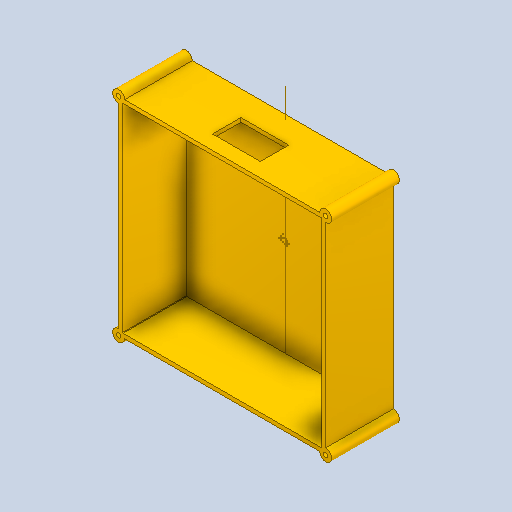
# Autodesk Inventor part: PS-01
Saved by Autodesk Inventor 2022 (Build 260153000, 153)
## iProperties
Company: El Camino College
Created: 2023-06-09
Part Number: PS-01
Material: Aluminum 6061(1)
Document SubType Name: Modeling
Designer: Edgar Tejada
Density: 2.7 g/cm^3
Appearance: Aluminum - Flat(1)
Mass: 533.78 g
Surface Area: 1266.21 cm^2
Volume: 197.696 cm^3
Author: Edgar Tejada
Title: Panel Shell
Autodesk Inventor part; units mm, degrees
ref_plane "YZ Plane" through (0, 0, 0) normal (1, 0, 0) x (0, 1, 0)
ref_plane "XZ Plane" through (0, 0, 0) normal (0, 1, 0) x (-1, 0, 0)
ref_plane "XY Plane" through (0, 0, 0) normal (0, 0, 1) x (1, 0, 0)
sketch "Sketch1" plane through (0, 0, 0) normal (0, 0, 1) x (1, 0, 0)
  line L0 (-79.375, 79.375) -> (79.375, 79.375)
  line L1 (79.375, 79.375) -> (79.375, -79.375)
  line L2 (79.375, -79.375) -> (-79.375, -79.375)
  line L3 (-79.375, -79.375) -> (-79.375, 79.375)
  line L4 (-79.375, 79.375) -> (79.375, -79.375) construction
  line L5 (79.375, 79.375) -> (-79.375, -79.375) construction
  point P0 (0, 0)
  dimension "d0" = 158.75
  constraints: 12 end point, 2 midpoint, 2 parallel, 2 perpendicular, 1 horizontal
  measures "d0" distance of L2.end L0.start
extrude "Extrusion1" add sketch "Sketch1" along normal blind 50.8
shell "Shell1" thickness 3.175 outward yes removed faces 1 at (-26.4583, 26.4583, 50.8)
sketch "Sketch2" plane through (0, 0, 0) normal (0, 0, 1) x (1, 0, 0)
  line L0 (-82.55, 82.55) -> (-82.55, -82.55) projected
  circle A0 centre (-82.55, 82.55) radius 4.7752
  line L1 (82.55, -82.55) -> (82.55, 82.55) projected
  circle A1 centre (82.55, 82.55) radius 4.7752
  line L2 (-82.55, -82.55) -> (82.55, -82.55) projected
  circle A2 centre (82.55, -82.55) radius 4.7752
  circle A3 centre (-82.55, -82.55) radius 4.7752
  point P0 (0, 0)
  dimension "d4" = 9.5504
  constraints: 4 centre point, 3 equal radius, 2 coincident
  measures "d4" diameter of A0
extrude "Extrusion2" add sketch "Sketch2" along normal blind 50.8 and the other way blind 3.175
sketch "Sketch3" plane through (0, 0, 50.8) normal (0, 0, 1) x (1, 0, 0)
  line L0 (-82.55, 77.7748) -> (-82.55, -77.7748) projected
  circle A0 centre (-82.55, -82.55) radius 1.7996
  circle A1 centre (82.55, 82.55) radius 1.7996
  line L1 (-77.7748, -82.55) -> (77.7748, -82.55) projected
  circle A2 centre (82.55, -82.55) radius 1.7996
  circle A3 centre (-82.55, 82.55) radius 1.7996
  point P0 (0, 0)
  dimension "d9" = 3.5992
  constraints: 4 centre point, 3 equal radius, 1 coincident
  measures "d9" diameter of A2
extrude "Extrusion3" cut sketch "Sketch3" along normal mid plane 107.95
sketch "Sketch4" plane through (-77.7748, 82.55, -3.175) normal (0, 1, 0) x (1, 0, 0)
  line L0 (58.7248, -19.939) -> (96.8248, -19.939)
  line L1 (96.8248, -19.939) -> (96.8248, -42.545)
  line L2 (96.8248, -42.545) -> (58.7248, -42.545)
  line L3 (58.7248, -42.545) -> (58.7248, -19.939)
  line L4 (58.7248, -19.939) -> (96.8248, -42.545) construction
  line L5 (96.8248, -19.939) -> (58.7248, -42.545) construction
  line L6 (155.5496, -53.975) -> (0, -53.975) projected
  point P0 (77.7748, -3.175)
  point P1 (77.7748, -31.242)
  point P2 (77.7748, -31.242)
  point P3 (160.9128, -53.975)
  point P4 (-0.588, -53.975)
  dimension "d12" = 38.1
  dimension "d13" = 22.606
  dimension "d14" = 11.43
  constraints: 12 end point, 3 midpoint, 2 parallel, 1 horizontal, 1 perpendicular, 1 vertical alignment
  measures "d12" distance of L0.start L0.end
  measures "d13" distance of L0.end L1.end
  measures "d14" distance between parallel lines of L2 L6
extrude "Extrusion4" cut sketch "Sketch4" against normal up to next
body "Solid1"
